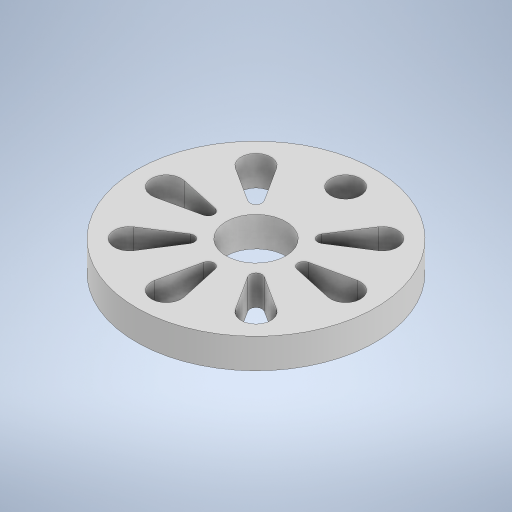
# Autodesk Inventor part: zebatka_mid
Saved by Autodesk Inventor 2024 (Build 280153000, 153)
## iProperties
Created: 2023-10-15
Part Number: zebatka_mid
Material: Generic
Document SubType Name: Modeling
Designer: Piter
Density: 1 g/cm^3
Appearance: Default
Author: Piter
Autodesk Inventor part; units mm, degrees
ref_plane "YZ Plane" through (0, 0, 0) normal (1, 0, 0) x (0, 1, 0)
ref_plane "XZ Plane" through (0, 0, 0) normal (0, 1, 0) x (-1, 0, 0)
ref_plane "XY Plane" through (0, 0, 0) normal (0, 0, 1) x (1, 0, 0)
sketch "Sketch1" plane through (0, 0, 0) normal (0, 1, 0) x (-1, 0, 0)
  circle A0 centre (0, 0) radius 20
  circle A1 centre (0, 0) radius 5
  line L0 (0, 0) -> (0, -15)
  circle A2 centre (0, -15) radius 2.5
  line L1 (0, 0) -> (20, 0)
  line L2 (0, 0) -> (15, 0)
  arc A3 (14.4643, -2.4419) -> (14.4643, 2.4419) centre (15, 0) ccw
  line L3 (15, 0) -> (8, 0)
  arc A4 (7.7857, 0.9768) -> (7.7857, -0.9768) centre (8, 0) ccw
  line L4 (14.4643, 2.4419) -> (7.7857, 0.9768)
  line L5 (7.7857, -0.9768) -> (14.4643, -2.4419)
  arc A5 (11.9545, 8.5011) -> (8.5011, 11.9545) centre (10.6066, 10.6066) ccw
  line L6 (10.6066, 10.6066) -> (5.6569, 5.6569)
  line L7 (8.5011, 11.9545) -> (4.8146, 6.196)
  line L8 (6.196, 4.8146) -> (11.9545, 8.5011)
  arc A6 (4.8146, 6.196) -> (6.196, 4.8146) centre (5.6569, 5.6569) ccw
  arc A7 (2.4419, 14.4643) -> (-2.4419, 14.4643) centre (0, 15) ccw
  line L9 (0, 15) -> (0, 8)
  line L10 (-2.4419, 14.4643) -> (-0.9768, 7.7857)
  line L11 (0.9768, 7.7857) -> (2.4419, 14.4643)
  arc A8 (-0.9768, 7.7857) -> (0.9768, 7.7857) centre (0, 8) ccw
  arc A9 (-8.5011, 11.9545) -> (-11.9545, 8.5011) centre (-10.6066, 10.6066) ccw
  line L12 (-10.6066, 10.6066) -> (-5.6569, 5.6569)
  line L13 (-11.9545, 8.5011) -> (-6.196, 4.8146)
  line L14 (-4.8146, 6.196) -> (-8.5011, 11.9545)
  arc A10 (-6.196, 4.8146) -> (-4.8146, 6.196) centre (-5.6569, 5.6569) ccw
  arc A11 (-14.4643, 2.4419) -> (-14.4643, -2.4419) centre (-15, 0) ccw
  line L15 (-15, 0) -> (-8, 0)
  line L16 (-14.4643, -2.4419) -> (-7.7857, -0.9768)
  line L17 (-7.7857, 0.9768) -> (-14.4643, 2.4419)
  arc A12 (-7.7857, -0.9768) -> (-7.7857, 0.9768) centre (-8, 0) ccw
  arc A13 (-11.9545, -8.5011) -> (-8.5011, -11.9545) centre (-10.6066, -10.6066) ccw
  line L18 (-10.6066, -10.6066) -> (-5.6569, -5.6569)
  line L19 (-8.5011, -11.9545) -> (-4.8146, -6.196)
  line L20 (-6.196, -4.8146) -> (-11.9545, -8.5011)
  arc A14 (-4.8146, -6.196) -> (-6.196, -4.8146) centre (-5.6569, -5.6569) ccw
  arc A15 (-2.4419, -14.4643) -> (2.4419, -14.4643) centre (0, -15) ccw
  line L21 (0, -15) -> (0, -8)
  line L22 (2.4419, -14.4643) -> (0.9768, -7.7857)
  line L23 (-0.9768, -7.7857) -> (-2.4419, -14.4643)
  arc A16 (0.9768, -7.7857) -> (-0.9768, -7.7857) centre (0, -8) ccw
  arc A17 (8.5011, -11.9545) -> (11.9545, -8.5011) centre (10.6066, -10.6066) ccw
  line L24 (10.6066, -10.6066) -> (5.6569, -5.6569)
  line L25 (11.9545, -8.5011) -> (6.196, -4.8146)
  line L26 (4.8146, -6.196) -> (8.5011, -11.9545)
  arc A18 (6.196, -4.8146) -> (4.8146, -6.196) centre (5.6569, -5.6569) ccw
  dimension "d0" = 40
  dimension "d1" = 10
  dimension "d2" = 15
  dimension "d3" = 5
  dimension "d4" = 15
  dimension "d5" = 5
  dimension "d6" = 7
  dimension "d7" = 2
  dimension "d10" = 360
  constraints: 54 end point, 32 point on circle, 19 coincident, 18 centre point, 4 tangent, 2 point on line, 1 horizontal, 1 horizontal alignment, 1 vertical, 107 other
  measures "d1" diameter of A1
  measures "d2" distance of L0.start L0.end
  measures "d3" diameter of A2
  measures "d4" distance of L0.start L2.end
  measures "d5" diameter of A3
  measures "d6" distance of L3.start L3.end
  measures "d7" diameter of A4
extrude "Extrusion1" add sketch "Sketch1" along normal blind 5 contours A0 | A16 L22 A2 L0 | L0 A2 L23 A16
body "Solid1"
